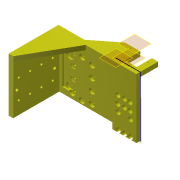
# Autodesk Inventor part: cellSTORM_Lasermount_v0
Saved by Autodesk Inventor 2019 (Build 230136000, 136)
## iProperties
Created: 2019-10-29
Part Number: cellSTORM_Lasermount_v0
Material: Generic
Document SubType Name: Modeling
Designer: diederichbenedict
Density: 1 g/cm^3
Appearance: Smooth - Yellow
Author: diederichbenedict
Autodesk Inventor part; units mm, degrees
ref_plane "YZ Plane" through (0, 0, 0) normal (1, 0, 0) x (0, 1, 0)
ref_plane "XZ Plane" through (0, 0, 0) normal (0, 1, 0) x (-1, 0, 0)
ref_plane "Work Plane1" through (0, 0, 0) normal (0, 0, 1) x (1, 0, 0)
sketch "Sketch1" plane through (0, 0, 0) normal (0, 0, 1) x (1, 0, 0)
  circle A0 centre (23.5, 33) radius 1 construction
  circle A1 centre (23.5, 43) radius 1 construction
  circle A2 centre (24, 3) radius 1 construction
  circle A3 centre (8, 3) radius 1 construction
  circle A4 centre (16, 33) radius 1 construction
  circle A5 centre (16, 43) radius 1 construction
  circle A6 centre (7.5, 43) radius 1 construction
  circle A7 centre (7.5, 33) radius 1.0474 construction
  circle A8 centre (16, 3) radius 1 construction
  line L0 (32, 0) -> (0, 0) construction
  line L1 (32, 0) -> (32, 48) construction
  line L2 (0, 48) -> (32, 48) construction
  line L3 (0, 0) -> (0, 48) construction
  line L4 (7.5277, 79) -> (26, 79) construction
  line L5 (26, 78) -> (7.5277, 78) construction
  line L6 (32, 0) -> (0, 0)
  line L7 (0, 0) -> (0, 79)
  line L8 (0, 79) -> (32, 79)
  line L9 (32, 79) -> (32, 0)
  constraints: 8 end point, 2 parallel, 1 horizontal, 1 perpendicular
ref_plane "Work Plane2" through (-70, 8, 5) normal (0, 0, 1) x (1, 0, 0)
ref_plane "Work Plane3" through (-91.5217, 38, 0) normal (0, 0, 1) x (0, 1, 0)
sketch "Sketch2" plane through (-91.5217, 38, 0) normal (0, 0, 1) x (0, 1, 0)
  line L0 (28, 30) -> (30, 28) construction
  line L1 (28, 30) -> (-28, 30) construction
  line L2 (-30, 28) -> (-28, 30) construction
  line L3 (-30, 28) -> (-30, -28) construction
  line L4 (-28, -30) -> (-30, -28) construction
  line L5 (-28, -30) -> (28, -30) construction
  line L6 (30, -28) -> (28, -30) construction
  line L7 (30, -28) -> (30, 28) construction
  circle A0 centre (-17.5, -17.5) radius 1.95 construction
  circle A1 centre (17.5, 17.5) radius 1.95 construction
  circle A2 centre (17.5, -17.5) radius 1.95 construction
  circle A3 centre (-17.5, 17.5) radius 1.95 construction
  circle A4 centre (0, 0) radius 7.5 construction
  line L8 (-38, -40) -> (41, -40) construction
  line L9 (-38, -72) -> (-38, -40) construction
  line L10 (41, -72) -> (-38, -72) construction
  line L11 (41, -40) -> (41, -72) construction
  line L12 (41, -40) -> (-30, -40)
  line L13 (-30, -40) -> (-30, 30)
  line L14 (-30, 30) -> (41, 30)
  line L15 (41, 30) -> (41, -40)
  line L16 (41, -72) -> (-38, -72) projected
  line L17 (41, -40) -> (-38, -40)
  line L18 (-38, -40) -> (-38, -72)
  line L19 (-38, -72) -> (41, -72)
  line L20 (41, -72) -> (41, -40)
  point P0 (-38, -91.5217)
  point P1 (41, -50.5)
  constraints: 16 end point, 4 parallel, 2 horizontal, 2 perpendicular, 1 point on line, 1 other
extrude "Extrusion2" add sketch "Sketch2" along normal blind 5
sketch "Sketch3" plane through (-91.5217, 38, 5) normal (0, 0, 1) x (1, 0, 0)
  line L0 (40, -30) -> (40, -38) projected
  line L1 (40, -38) -> (72, -38) projected
  line L2 (72, -38) -> (72, 41) projected
  line L3 (72, 41) -> (-30, 41) projected
  line L4 (-30, 41) -> (-30, -30) projected
  line L5 (-30, -30) -> (40, -30) projected
  circle A0 centre (48, -35) radius 1 projected
  circle A1 centre (64, -35) radius 1 projected
  circle A2 centre (63.5, 5) radius 1 projected
  circle A3 centre (63.5, -5) radius 1 projected
  circle A4 centre (47.5, -5) radius 1.0474 projected
  circle A5 centre (47.5, 5) radius 1 projected
  arc A6 (64.5499, 87.15) -> (61.0499, 90.65) centre (61.0499, 87.15) ccw projected
  line L6 (2.1699, 90.65) -> (61.0499, 90.65) projected
  arc A7 (2.1699, 90.65) -> (-1.3301, 87.15) centre (2.1699, 87.15) ccw projected
  line L7 (-1.3301, -52.85) -> (-1.3301, 87.15) projected
  arc A8 (-1.3301, -52.85) -> (2.1699, -56.35) centre (2.1699, -52.85) ccw projected
  line L8 (61.0499, -56.35) -> (2.1699, -56.35) projected
  arc A9 (61.0499, -56.35) -> (64.5499, -52.85) centre (61.0499, -52.85) ccw projected
  line L9 (64.5499, 87.15) -> (64.5499, -52.85) projected
  circle A10 centre (56, 5) radius 1 projected
  circle A11 centre (56, -5) radius 1 projected
  circle A12 centre (56, -35) radius 1 projected
  circle A13 centre (47.35, -14.5) radius 1.4 projected
  circle A14 centre (63.65, -14.5) radius 1.4 projected
  point P0 (91.5217, -38)
hole "Hole1" at (-44.0217, 43, 5) at (-35.5217, 43, 5) at (-28.0217, 43, 5) at (-28.0217, 33, 5) at (-35.5217, 33, 5) at (-44.0217, 33, 5) at (-43.5217, 3, 5) at (-35.5217, 3, 5) at (-27.5217, 3, 5) at (-44.1717, 23.5, 5) at (-27.8717, 23.5, 5) direction (0, 0, -1) diameter 3.6 depth 12 tip angle 118 counterbore diameter 6.5 counterbore depth 4
sketch "Sketch4" plane through (-91.5217, 38, 5) normal (0, 0, 1) x (1, 0, 0)
  circle A0 centre (13.1592, 7.4996) radius 3 construction
  circle A1 centre (13, -22.5) radius 3 construction
  circle A2 centre (-12.92, -7.3622) radius 3 construction
  circle A3 centre (-12.7608, 22.6373) radius 3 construction
  circle A4 centre (-12.8404, 7.6376) radius 3 construction
  circle A5 centre (-12.9996, -22.362) radius 3 construction
  circle A6 centre (13.0796, -7.5002) radius 3 construction
  circle A7 centre (13.2388, 22.4994) radius 3 construction
  circle A8 centre (-0.0131, -24.931) radius 1.95 construction
  circle A9 centre (0.2523, 25.0683) radius 1.95 construction
  line L0 (-30.0286, -27.7717) -> (-28.0392, -29.7823) construction
  line L1 (-28.0392, -29.7823) -> (27.96, -30.0795) construction
  line L2 (27.96, -30.0795) -> (29.9706, -28.0901) construction
  line L3 (29.9706, -28.0901) -> (30.2678, 27.9091) construction
  line L4 (30.2678, 27.9091) -> (28.2784, 29.9197) construction
  line L5 (28.2784, 29.9197) -> (-27.7208, 30.2168) construction
  line L6 (-27.7208, 30.2168) -> (-29.7314, 28.2275) construction
  line L7 (-29.7314, 28.2275) -> (-30.0286, -27.7717) construction
  point P0 (-17.5, -17.5)
  point P1 (17.5, -17.5)
  point P2 (17.5, 17.5)
  point P3 (-17.5, 17.5)
hole "Hole2" at (-104.2825, 60.6373, 5) at (-104.3621, 45.6376, 5) at (-104.4417, 30.6378, 5) at (-104.5213, 15.638, 5) at (-91.5347, 13.069, 5) at (-91.2694, 63.0683, 5) at (-78.2829, 60.4994, 5) at (-78.3625, 45.4996, 5) at (-78.4421, 30.4998, 5) at (-78.5217, 15.5, 5) direction (0, 0, -1) diameter 3.1 depth 12 tip angle 118 counterbore diameter 8 counterbore depth 3
ref_plane "Work Plane4" through (0, 79, 0) normal (0, 1, 0) x (1, 0, 0)
sketch "Sketch5" plane through (0, 79, 0) normal (0, 1, 0) x (1, 0, 0)
  arc A0 (0.1445, 22.7) -> (-0.8555, 23.7) centre (-0.8555, 22.7) ccw construction
  line L0 (-0.8555, 23.7) -> (-4, 23.7) construction
  line L1 (-4, 23.7) -> (-4, -2) construction
  line L2 (-4, -2) -> (5.5277, -2) construction
  arc A1 (5.5277, -2) -> (6.5277, -1) centre (5.5277, -1) ccw construction
  line L3 (6.5277, -1) -> (6.5277, 0.8624) construction
  arc A2 (7.5277, 1.8624) -> (6.5277, 0.8624) centre (7.5277, 0.8624) ccw construction
  line L4 (7.5277, 1.8624) -> (26, 1.8624) construction
  line L5 (26, 1.8624) -> (26, 13.397) construction
  arc A3 (27, 14.397) -> (26, 13.397) centre (27, 13.397) ccw construction
  line L6 (27, 14.397) -> (28, 14.397) construction
  arc A4 (28, 14.397) -> (29, 15.397) centre (28, 15.397) ccw construction
  line L7 (29, 15.397) -> (29, 17.9624) construction
  arc A5 (29, 17.9624) -> (28, 18.9624) centre (28, 17.9624) ccw construction
  line L8 (28, 18.9624) -> (1.1445, 18.9624) construction
  arc A6 (0.1445, 19.9624) -> (1.1445, 18.9624) centre (1.1445, 19.9624) ccw construction
  line L9 (0.1445, 19.9624) -> (0.1445, 22.7) construction
  line L10 (8.5, 17) -> (24, 17) construction
  line L11 (24, 17) -> (24, 3.5) construction
  line L12 (24, 3.5) -> (8.5, 3.5) construction
  line L13 (8.5, 3.5) -> (8.5, 17) construction
  circle A7 centre (-1.5, 21) radius 1 construction
  circle A8 centre (5, 0.5) radius 1 construction
  circle A9 centre (26.5, 16) radius 1 construction
  line L14 (-19.5217, 0) -> (-19.5217, -5) construction
  line L15 (-19.5217, 0) -> (-121.5217, 0) construction
  line L16 (-51.5217, 0) -> (-19.5217, 0) projected
  line L17 (-4, 23.7) -> (-19.5217, 23.7)
  line L18 (-19.5217, 23.7) -> (-19.5217, 0)
  line L19 (-19.5217, 0) -> (-4, 0)
  line L20 (-4, 0) -> (-4, 23.7)
  line L21 (8.5, 3.5) -> (24, 3.5)
  line L22 (24, 3.5) -> (24, 23.7)
  line L23 (24, 23.7) -> (8.5, 23.7)
  line L24 (8.5, 23.7) -> (8.5, 3.5)
  constraints: 16 end point, 4 parallel, 2 horizontal, 2 perpendicular, 1 point on line
extrude "Extrusion3" [suppressed]
sketch "Sketch6" plane through (-121.5217, 8, 0) normal (-1, 0, 0) x (0, 0, 1)
  circle A0 centre (61, 30) radius 1.95 projected
  circle A1 centre (36, 55) radius 1.95 projected
  circle A2 centre (11, 55) radius 1.95 projected
  circle A3 centre (61, 5) radius 1.95 projected
  circle A4 centre (11, 5) radius 1.95 projected
  circle A5 centre (61, 55) radius 1.95 projected
  circle A6 centre (36, 5) radius 1.95 projected
  circle A7 centre (11, 30) radius 1.95 projected
  line L0 (66, 58) -> (64, 60) projected
  line L1 (64, 60) -> (8, 60) projected
  line L2 (8, 60) -> (6, 58) projected
  line L3 (6, 58) -> (6, 2) projected
  line L4 (6, 2) -> (8, 0) projected
  line L5 (8, 0) -> (64, 0) projected
  line L6 (64, 0) -> (66, 2) projected
  line L7 (66, 2) -> (66, 58) projected
  line L8 (0, 71) -> (0, 0) projected
  line L9 (0, 0) -> (5, 0) projected
  line L10 (5, 71) -> (5, 0) projected
  line L11 (0, 71) -> (5, 71) projected
  line L12 (66, 0) -> (0, 0)
  line L13 (0, 0) -> (0, 71)
  line L14 (0, 71) -> (66, 71)
  line L15 (66, 71) -> (66, 0)
  circle A8 centre (58.5, 43) radius 1.45 projected
  circle A9 centre (43.5, 43) radius 1.45 projected
  circle A10 centre (28.5, 43) radius 1.45 projected
  circle A11 centre (13.5, 43) radius 1.45 projected
  circle A12 centre (13.5, 17) radius 1.45 projected
  circle A13 centre (28.5, 17) radius 1.45 projected
  circle A14 centre (43.5, 17) radius 1.45 projected
  circle A15 centre (58.5, 17) radius 1.45 projected
  point P0 (0, -8)
  constraints: 8 end point, 2 parallel, 1 horizontal, 1 perpendicular, 1 point on line
extrude "Extrusion4" add sketch "Sketch6" along normal blind 6 contours A1 | A2 | A3 | A4 | A5 | A6 | L7 L6 L5 L4 L3 L2 L1 L0 | L0 L1 L2 L3 L4 L12 L10 L14 L15 | L15 L12 L6 | L10 L9 L8 L11
ref_plane "Work Plane6" through (-4, 79, -28.7) normal (0, 1, 0) x (1, 0, 0)
sketch "Sketch7" plane through (-4, 79, -28.7) normal (0, 1, 0) x (1, 0, 0)
  line L0 (-117.5217, -94.7) -> (-31, -33.7)
  line L1 (-28.2146, -29.9678) -> (0, -33.7)
  line L2 (-37.7992, -28.7) -> (-28.2146, -29.9678)
  line L3 (-7.7257, -5.1) -> (-37.7992, -28.7)
  line L4 (-7.7257, -5.1) -> (0, -4.9497)
  line L5 (0, -4.9497) -> (0, -33.7)
  line L6 (-15.5217, -28.7) -> (-123.5217, -28.7) projected
  line L7 (-37.7992, -28.7) -> (0, -33.7)
  line L8 (-47.5217, -28.7) -> (-123.5217, -28.7) projected
  line L9 (-123.5217, -28.7) -> (-37.7992, -28.7)
  line L10 (-31, -33.7) -> (-31, -29.5994)
  line L11 (-117.5217, -94.7) -> (-123.5217, -94.7) projected
  line L12 (-123.5217, -28.7) -> (-123.5217, -94.7)
  line L13 (-123.5217, -94.7) -> (-117.5217, -94.7)
  point P0 (0, -28.7)
  constraints: 22 end point, 3 vertical, 2 collinear, 1 horizontal, 1 point on line, 2 other
extrude "Extrusion5" add sketch "Sketch7" against normal blind 6
sketch "Sketch8" plane through (-91.5217, 38, 5) normal (0, 0, 1) x (1, 0, 0)
  line L0 (0, 28) -> (-10, 28) construction
  line L1 (0, -28) -> (0, 28) construction
  line L2 (-10, -28) -> (0, -28) construction
  line L3 (-10, -28) -> (-10, 28) construction
  line L4 (-10, -28) -> (-10, 28) construction
  line L5 (-10, -28) -> (-20, -28) construction
  line L6 (-20, 28) -> (-20, -28) construction
  line L7 (-10, 28) -> (-20, 28) construction
  circle A0 centre (-17.5, -17.5) radius 2.1 projected
  circle A1 centre (-17.5, 17.5) radius 2.1 projected
  circle A2 centre (-17.5, -17.5) radius 5.1
  circle A3 centre (-17.5, 17.5) radius 5.1
  point P0 (91.5217, -38)
  dimension "d28" = 3
  dimension "d29" = 3
  constraints: 2 centre point
  measures "d28" radial gap between concentric circles of A0 A2
  measures "d29" radial gap between concentric circles of A1 A3
extrude "Extrusion6" cut sketch "Sketch8" against normal blind 4 contours A0 | A1 | A2 | A3
sketch "Sketch9" plane through (-91.5217, 38, 5) normal (0, 0, 1) x (1, 0, 0)
  line L0 (-29.973, -22.5) -> (-7.973, -22.5) construction
  line L1 (-7.973, -22.5) -> (-7.973, 23.5) construction
  line L2 (-7.973, 23.5) -> (-29.973, 23.5) construction
  line L3 (-29.973, 23.5) -> (-29.973, -22.5) construction
  line L4 (-30, -30) -> (40, -30) construction
  line L5 (-7.973, -22.5) -> (-25.973, -22.5)
  line L6 (-25.973, -22.5) -> (-25.973, 23.5)
  line L7 (-25.973, 23.5) -> (-7.973, 23.5)
  line L8 (-7.973, 23.5) -> (-7.973, -22.5)
  point P0 (91.5217, -38)
  dimension "d32" = 22
  dimension "d33" = 46
  dimension "d34" = 7.5
  dimension "d35" = 18
  constraints: 16 end point, 4 parallel, 2 horizontal, 2 perpendicular, 1 point on line
  measures "d32" distance of L2.end L1.end
  measures "d33" distance of L1.end L0.end
  measures "d34" distance between parallel lines of L0 L4
  measures "d35" distance of L6.end L7.end
extrude "Extrusion7" cut sketch "Sketch9" against normal blind 2
ref_plane "Work Plane5" through (8.5, 79, -8.5) normal (0, 1, 0) x (1, 0, 0)
sketch "Sketch10" plane through (8.5, 79, -8.5) normal (0, 1, 0) x (1, 0, 0)
  circle A0 centre (-10, 12.5) radius 1 projected
  circle A1 centre (-3.5, -8) radius 1 projected
  circle A2 centre (18, 7.5) radius 1 projected
  point P0 (18, 12.5)
  point P1 (-3.5, -3)
  point P2 (-10, 17.5)
hole "Hole3" at (5, 79, -5.5) at (-1.5, 79, -21) at (26.5, 79, -16) at (5, 79, -0.5) direction (0, -1, 0) diameter 1.2 depth 10 tip angle 118
body "Solid1"
